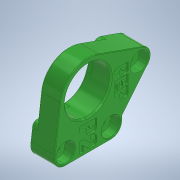
# Autodesk Inventor part: X-Axis Motor Support
Saved by Autodesk Inventor 2020 (Build 240168000, 168)
## iProperties
Created: 2019-09-17
Part Number: X-Axis Motor Support
Material: Generic
Document SubType Name: Modeling
Designer: pepd9
Density: 1 g/cm^3
Appearance: Smooth - Dark Forest Green
Author: pepd9
Autodesk Inventor part; units mm, degrees
ref_plane "YZ Plane" through (0, 0, 0) normal (1, 0, 0) x (0, 1, 0)
ref_plane "XZ Plane" through (0, 0, 0) normal (0, 1, 0) x (-1, 0, 0)
ref_plane "XY Plane" through (0, 0, 0) normal (0, 0, 1) x (1, 0, 0)
sketch "Sketch1" plane through (0, 0, 0) normal (1, 0, 0) x (0, 1, 0)
  circle A0 centre (0, 0) radius 8
  circle A1 centre (0, 0) radius 10
  dimension "d0" = 16
  dimension "d1" = 20
  constraints: 2 centre point, 2 coincident
  measures "d0" diameter of A0
  measures "d1" diameter of A1
extrude "Extrusion1" add sketch "Sketch1" along normal blind 6
sketch "Sketch2" plane through (0, 0, 0) normal (-1, 0, 0) x (0, 0, 1)
  circle A0 centre (0, 0) radius 8
  circle A1 centre (-18, 0) radius 2.75 construction
  circle A2 centre (-18, 0) radius 4
  circle A3 centre (0, 0) radius 10
  circle A4 centre (-18, 0) radius 1.5 construction
  line L0 (-19.5, 3.708099) -> (-3.736025, 9.275889)
  circle A5 centre (0, 0) radius 10
  line L1 (-12.888145, -9.569739) -> (-10.705089, -10.830127) construction
  line L2 (10.373932, -10.830127) -> (12.998008, -9.315116) construction
  circle A6 centre (-8, -15) radius 1.5 construction
  circle A7 centre (8, -15) radius 1.5 construction
  circle A8 centre (8, -15) radius 2.75 construction
  circle A9 centre (-8, -15) radius 2.75 construction
  circle A10 centre (-8, -15) radius 4
  circle A11 centre (8, -15) radius 4
  line L3 (-12, -15) -> (-12, -13.5)
  line L4 (11.832818, -13.855665) -> (9.920905, 1.255246)
  line L5 (8, -19) -> (-8, -19)
  line L6 (-12, -13.5) -> (-20.414736, -3.188895)
  point P0 (9.920905, 1.255246)
  point P1 (-3.736025, 9.275889)
  dimension "d4" = 5.5
  dimension "d5" = 8
  dimension "d6" = 18
  dimension "d7" = 3
  dimension "d8" = 3
  dimension "d9" = 3
  dimension "d10" = 5.5
  dimension "d11" = 5.5
  dimension "d12" = 8
  dimension "d13" = 8
  dimension "d14" = 15
  dimension "d15" = 8
  dimension "d16" = 8
  constraints: 10 end point, 9 centre point, 9 coincident, 8 point on circle, 2 tangent, 1 horizontal alignment, 1 vertical
  measures "d4" diameter of A1
  measures "d5" diameter of A2
  measures "d6" distance of point (0, 0) A1.centre
  measures "d7" diameter of A4
  measures "d8" diameter of A6
  measures "d9" diameter of A7
  measures "d10" diameter of A8
  measures "d11" diameter of A9
  measures "d12" diameter of A10
  measures "d13" diameter of A11
  measures "d14" vertical distance of A6.centre point (0, 0)
  measures "d15" horizontal distance of point (0, 0) A8.centre
  measures "d16" horizontal distance of point (0, 0) A6.centre
extrude "Extrusion2" add sketch "Sketch2" against normal blind 6 contours A2 | A2 L0 A3 L4 A11 L5 A10 L3 L6 | A10 | A11
sketch "Sketch3" plane through (6, 0, 0) normal (1, 0, 0) x (0, 0, -1)
  arc A0 (20.414736, -3.188895) -> (19.5, 3.708099) centre (18, 0) ccw
  arc A1 (8, -19) -> (12, -15) centre (8, -15) ccw
  arc A2 (-11.832818, -13.855665) -> (-8, -19) centre (-8, -15) ccw
  point P0 (0, 0)
hole "Hole1" at (6, 0, -18) at (6, -15, -8) at (6, -15, 8) direction (-1, 0, 0) diameter 3.2 end through all counterbore diameter 6.5 counterbore depth 2 clearance for "Socket Head Cap Screw" size "M3" standard "Ansi Metric M Profile"
sketch "Sketch4" plane through (6, 0, 0) normal (1, 0, 0) x (0, 0, -1)
  circle A0 centre (8, -15) radius 3.25
  circle A1 centre (18, 0) radius 3.25
  circle A2 centre (-8, -15) radius 3.25
  arc A3 (3.736025, 9.275889) -> (-9.920905, 1.255246) centre (0, 0) ccw
  line L0 (-9.920905, 1.255246) -> (-11.832818, -13.855665)
  arc A4 (-11.832818, -13.855665) -> (-8, -19) centre (-8, -15) ccw
  line L1 (-8, -19) -> (8, -19)
  arc A5 (8, -19) -> (12, -15) centre (8, -15) ccw
  line L2 (12, -15) -> (12, -13.5)
  line L3 (12, -13.5) -> (20.414736, -3.188895)
  arc A6 (20.414736, -3.188895) -> (19.5, 3.708099) centre (18, 0) ccw
  line L4 (19.5, 3.708099) -> (3.736025, 9.275889)
  circle A7 centre (0, 0) radius 8
  circle A8 centre (0, 0) radius 4
  dimension "d26" = 8
  constraints: 1 centre point, 1 coincident
  measures "d26" diameter of A8
extrude "Extrusion3" add sketch "Sketch4" along normal blind 1 contours L4 A6 L3 L2 A5 L1 A4 L0 A3 | A7
sketch "Sketch5" plane through (0, 0, 0) normal (-1, 0, 0) x (0, 0, 1)
  circle A0 centre (-8, -15) radius 1.6
  circle A1 centre (-18, 0) radius 1.6
  circle A2 centre (8, -15) radius 1.6
  arc A3 (9.920905, 1.255246) -> (-3.736025, 9.275889) centre (0, 0) ccw
  line L0 (-3.736025, 9.275889) -> (-19.5, 3.708099)
  arc A4 (-19.5, 3.708099) -> (-20.414736, -3.188895) centre (-18, 0) ccw
  line L1 (-20.414736, -3.188895) -> (-12, -13.5)
  line L2 (-12, -13.5) -> (-12, -15)
  arc A5 (-12, -15) -> (-8, -19) centre (-8, -15) ccw
  line L3 (-8, -19) -> (8, -19)
  arc A6 (8, -19) -> (11.832818, -13.855665) centre (8, -15) ccw
  line L4 (11.832818, -13.855665) -> (9.920905, 1.255246)
  circle A7 centre (0, 0) radius 8
  circle A8 centre (0, 0) radius 8
  line L5 (0, -8) -> (11.091928, -8)
  line L6 (11.832818, -13.855665) -> (9.920905, 1.255246)
  line L7 (-7.667515, -2.282371) -> (-10.979812, 6.717405)
  constraints: 4 end point, 2 point on circle, 2 point on line, 1 horizontal, 1 tangent
ref_plane "Work Plane1" through (-3.5, -20.915116, -29.665578) normal (1, 0, 0) x (0, 1, 0)
extrude "Extrusion4" add sketch "Sketch5" along normal blind 1.8 contours L4 A6 L3 A5 L2 L1 A4 L0 L7 A7 L5
fillet "Fillet1" radius 2 2 edges at (-0.9, -8, 11.0919) (-0.9, 6.7174, -10.9798)
chamfer "Chamfer1" distance 0.5 angle 45 13 edges at (-1.8, 0.5259, -21.9653) (-1.8, 4.8841, -16.1705) (-1.8, 5.9843, -11.3243) (-1.8, 1.2913, -8.9828) (-1.8, -6.4132, -4.7823) (-1.8, -8, 4.6645) (-1.8, -8.4997, 10.6515) (-1.8, -11.8023, 11.573) (-1.8, -17.3898, 11.2076) (-1.8, -19, 0) (-1.8, -17.8284, -10.8284) (-1.8, -14.25, -12) (-1.8, -8.3444, -16.2074)
chamfer "Chamfer2" distance 0.2 angle 45 12 edges at (7, 8.6229, 5.0642) (7, -6.3002, 10.8769) (7, 6.492, -11.618) (7, 0.5259, -21.9653) (7, -8.3444, -16.2074) (7, -17.8284, -10.8284) (7, -14.25, -12) (7, -19, 0) (7, -17.3898, 11.2076) (7, -15, 11.25) (7, 0, 4) (7, -15, -4.75)
chamfer "Chamfer3" distance 0.5 angle 45 5 edges at (0, -3.3724, 10.5064) (0, -8.8745, 11.2026) (0, 8.6229, 5.0642) (0, 7.9966, -7.3579) (0, 6.3887, -11.9104)
chamfer "Chamfer4" distance 0.5 angle 45 2 edges at (0, 4.7823, -6.4132) (0, 0, 8)
sketch "Sketch7" plane through (4, 0, -18) normal (1, 0, 0) x (0, 0, -1)
  circle A0 centre (0, 0) radius 3.25 projected
  circle A1 centre (0, 0) radius 1.6 projected
  circle A2 centre (-10, -15) radius 3.25 projected
  circle A3 centre (-10, -15) radius 1.6 projected
  circle A4 centre (-26, -15) radius 3.25 projected
  circle A5 centre (-26, -15) radius 1.6 projected
  line L0 (-3.25, 1.6) -> (3.25, 1.6)
  line L1 (3.25, 1.6) -> (3.25, -1.6)
  line L2 (3.25, -1.6) -> (-3.25, -1.6)
  line L3 (-3.25, -1.6) -> (-3.25, 1.6)
  line L4 (-3.25, 1.6) -> (3.25, -1.6) construction
  line L5 (3.25, 1.6) -> (-3.25, -1.6) construction
  line L6 (-13.25, -13.4) -> (-6.75, -13.4)
  line L7 (-6.75, -13.4) -> (-6.75, -16.6)
  line L8 (-6.75, -16.6) -> (-13.25, -16.6)
  line L9 (-13.25, -16.6) -> (-13.25, -13.4)
  line L10 (-13.25, -13.4) -> (-6.75, -16.6) construction
  line L11 (-6.75, -13.4) -> (-13.25, -16.6) construction
  line L12 (-29.25, -13.4) -> (-22.75, -13.4)
  line L13 (-22.75, -13.4) -> (-22.75, -16.6)
  line L14 (-22.75, -16.6) -> (-29.25, -16.6)
  line L15 (-29.25, -16.6) -> (-29.25, -13.4)
  line L16 (-29.25, -13.4) -> (-22.75, -16.6) construction
  line L17 (-22.75, -13.4) -> (-29.25, -16.6) construction
  point P0 (-18, 0)
  point P1 (-26, -16.6)
  point P2 (-23.171131, -16.6)
  point P3 (-23.171131, -13.4)
  point P4 (-26, -13.4)
  point P5 (-28.828869, -16.6)
  point P6 (-28.828869, -13.4)
  point P7 (-10, -16.6)
  point P8 (-7.171131, -16.6)
  point P9 (-7.171131, -13.4)
  point P10 (-10, -13.4)
  point P11 (-12.828869, -16.6)
  point P12 (-12.828869, -13.4)
  point P13 (-2.828869, -1.6)
  point P14 (0, -1.6)
  point P15 (0, 1.6)
  point P16 (-2.828869, 1.6)
  point P17 (2.828869, -1.6)
  point P18 (2.828869, 1.6)
  constraints: 36 end point, 6 midpoint, 6 parallel, 3 horizontal, 3 perpendicular
extrude "Extrusion6" cut sketch "Sketch7" against normal blind 0.4 contours A0 L2 A1 L0 | L0 A1 L2 A0 | A2 L8 A3 L6 | L6 A3 L8 A2 | A4 L14 A5 L12 | L12 A5 L14 A4
sketch "Sketch8" plane through (7, 0, 0) normal (1, 0, 0) x (0, 0, -1)
  circle A0 centre (0, 0) radius 8 projected
extrude "Extrusion7" cut sketch "Sketch8" against normal through all
chamfer "Chamfer5" distance 0.5 angle 45 1 edges at (7, 0, 8)
sketch "Sketch9" plane through (7, 0, 0) normal (1, 0, 0) x (0, 0, -1)
  line L0 (14.09513, 2.10245) -> (14.09513, -15.072793) construction
  line L1 (14.09513, -15.072793) -> (6.09513, -15.072793) construction
  line L2 (6.09513, -15.072793) -> (6.09513, 2.10245) construction
  line L3 (6.09513, 2.10245) -> (14.09513, 2.10245) construction
  line L4 (9.09513, 1.833994) -> (14.09513, 1.833994)
  line L5 (14.09513, 1.833994) -> (14.09513, -0.116043)
  spline S0 degree 2 poles (14.09513, -0.116043) (14.09513, -0.794642) (13.502289, -1.49934) (12.864705, -1.603739) knots 0 0 0 1 2 2 2
  spline S1 degree 2 poles (12.864705, -1.603739) (12.655906, -1.633568) (12.510492, -1.641025) (12.454563, -1.641025) knots 0 0 0 1 2 2 2
  spline S2 degree 2 poles (12.454563, -1.641025) (11.749865, -1.641025) (10.959411, -0.768542) (10.959411, 0.010728) knots 0 0 0 1 2 2 2
  line L6 (10.959411, 0.010728) -> (10.959411, 0.405955)
  line L7 (10.959411, 0.405955) -> (9.09513, 0.405955)
  line L8 (9.09513, 0.405955) -> (9.09513, 1.833994)
  spline S3 degree 2 poles (12.010865, 0.193427) (12.010865, 0.089027) (12.186107, -0.134686) (12.365078, -0.171972) knots 0 0 0 1 2 2 2
  spline S4 degree 2 poles (12.365078, -0.171972) (12.458292, -0.190615) (12.54032, -0.190615) knots 0 0 0 1 1 1
  spline S5 degree 2 poles (12.54032, -0.190615) (12.771491, -0.190615) (13.036219, 0.025642) (13.036219, 0.178513) knots 0 0 0 1 2 2 2
  line L9 (13.036219, 0.178513) -> (13.036219, 0.405955)
  line L10 (13.036219, 0.405955) -> (12.010865, 0.405955)
  line L11 (12.010865, 0.405955) -> (12.010865, 0.193427)
  line L12 (9.09513, -1.842367) -> (14.09513, -1.842367)
  line L13 (14.09513, -1.842367) -> (14.09513, -4.847587)
  line L14 (14.09513, -4.847587) -> (12.939276, -4.847587)
  line L15 (12.939276, -4.847587) -> (12.939276, -3.270406)
  line L16 (12.939276, -3.270406) -> (12.193564, -3.270406)
  line L17 (12.193564, -3.270406) -> (12.193564, -4.750645)
  line L18 (12.193564, -4.750645) -> (11.086182, -4.750645)
  line L19 (11.086182, -4.750645) -> (11.086182, -3.270406)
  line L20 (11.086182, -3.270406) -> (10.250984, -3.270406)
  line L21 (10.250984, -3.270406) -> (10.250984, -4.899787)
  line L22 (10.250984, -4.899787) -> (9.09513, -4.899787)
  line L23 (9.09513, -4.899787) -> (9.09513, -1.842367)
  line L24 (9.09513, -5.224172) -> (14.09513, -5.224172)
  line L25 (14.09513, -5.224172) -> (14.09513, -7.174209)
  spline S6 degree 2 poles (14.09513, -7.174209) (14.09513, -7.852807) (13.502289, -8.557505) (12.864705, -8.661905) knots 0 0 0 1 2 2 2
  spline S7 degree 2 poles (12.864705, -8.661905) (12.655906, -8.691733) (12.510492, -8.69919) (12.454563, -8.69919) knots 0 0 0 1 2 2 2
  spline S8 degree 2 poles (12.454563, -8.69919) (11.749865, -8.69919) (10.959411, -7.826707) (10.959411, -7.047438) knots 0 0 0 1 2 2 2
  line L26 (10.959411, -7.047438) -> (10.959411, -6.652211)
  line L27 (10.959411, -6.652211) -> (9.09513, -6.652211)
  line L28 (9.09513, -6.652211) -> (9.09513, -5.224172)
  spline S9 degree 2 poles (12.010865, -6.864738) (12.010865, -6.969138) (12.186107, -7.192852) (12.365078, -7.230137) knots 0 0 0 1 2 2 2
  spline S10 degree 2 poles (12.365078, -7.230137) (12.458292, -7.24878) (12.54032, -7.24878) knots 0 0 0 1 1 1
  spline S11 degree 2 poles (12.54032, -7.24878) (12.771491, -7.24878) (13.036219, -7.032524) (13.036219, -6.879653) knots 0 0 0 1 2 2 2
  line L29 (13.036219, -6.879653) -> (13.036219, -6.652211)
  line L30 (13.036219, -6.652211) -> (12.010865, -6.652211)
  line L31 (12.010865, -6.652211) -> (12.010865, -6.864738)
  point P0 (0, 0)
  constraints: 2 other
extrude "Extrusion8" cut sketch "Sketch9" against normal blind 0.6
sketch "Sketch10" plane through (7, 0, 0) normal (1, 0, 0) x (0, 0, -1)
  line L0 (3.056419, -9.325871) -> (3.056419, -19.630122) construction
  line L1 (3.056419, -19.630122) -> (-4.027101, -19.630122) construction
  line L2 (-4.027101, -19.630122) -> (-4.027101, -9.325871) construction
  line L3 (-4.027101, -9.325871) -> (3.056419, -9.325871) construction
  line L4 (-3.01517, -9.648019) -> (2.984831, -9.648019)
  line L5 (2.984831, -9.648019) -> (2.984831, -11.988064)
  spline S0 degree 2 poles (2.984831, -11.988064) (2.984831, -12.802381) (2.273421, -13.648019) (1.50832, -13.773298) knots 0 0 0 1 2 2 2
  spline S1 degree 2 poles (1.50832, -13.773298) (1.257761, -13.809093) (1.083264, -13.818041) (1.01615, -13.818041) knots 0 0 0 1 2 2 2
  spline S2 degree 2 poles (1.01615, -13.818041) (0.170513, -13.818041) (-0.778033, -12.771061) (-0.778033, -11.835938) knots 0 0 0 1 2 2 2
  line L6 (-0.778033, -11.835938) -> (-0.778033, -11.361665)
  line L7 (-0.778033, -11.361665) -> (-3.01517, -11.361665)
  line L8 (-3.01517, -11.361665) -> (-3.01517, -9.648019)
  spline S3 degree 2 poles (0.483712, -11.616699) (0.483712, -11.741979) (0.694003, -12.010435) (0.908768, -12.055178) knots 0 0 0 1 2 2 2
  spline S4 degree 2 poles (0.908768, -12.055178) (1.020625, -12.077549) (1.119059, -12.077549) knots 0 0 0 1 1 1
  spline S5 degree 2 poles (1.119059, -12.077549) (1.396464, -12.077549) (1.714137, -11.818041) (1.714137, -11.634596) knots 0 0 0 1 2 2 2
  line L9 (1.714137, -11.634596) -> (1.714137, -11.361665)
  line L10 (1.714137, -11.361665) -> (0.483712, -11.361665)
  line L11 (0.483712, -11.361665) -> (0.483712, -11.616699)
  spline S6 degree 2 poles (-3.01517, -13.997012) (-2.514051, -13.997012) (-1.838436, -14.122292) (-1.498391, -14.296788) knots 0 0 0 1 2 2 2
  spline S7 degree 2 poles (-1.498391, -14.296788) (-1.194141, -14.439965) (-0.710919, -14.833701) (-0.330606, -15.227437) knots 0 0 0 1 2 2 2
  line L12 (-0.330606, -15.227437) -> (0.152616, -15.697236)
  spline S8 degree 2 poles (0.152616, -15.697236) (0.613466, -16.108869) (1.011676, -16.310211) (1.347247, -16.310211) knots 0 0 0 1 2 2 2
  spline S9 degree 2 poles (1.347247, -16.310211) (1.463578, -16.310211) (1.620177, -16.28784) (1.69624, -16.25652) knots 0 0 0 1 2 2 2
  spline S10 degree 2 poles (1.69624, -16.25652) (1.924428, -16.158086) (1.924428, -15.974641) knots 0 0 0 1 1 1
  spline S11 degree 2 poles (1.924428, -15.974641) (1.924428, -15.934372) (1.866262, -15.755401) (1.553063, -15.621173) (1.168276, -15.621173) knots 0 0 0 1 2 3 3 3
  line L13 (1.168276, -15.621173) -> (0.908768, -15.621173)
  line L14 (0.908768, -15.621173) -> (0.908768, -14.019384)
  line L15 (0.908768, -14.019384) -> (1.213018, -14.014909)
  spline S12 degree 2 poles (1.213018, -14.014909) (1.825994, -14.014909) (2.573197, -14.408645) (2.819282, -14.865021) knots 0 0 0 1 2 2 2
  spline S13 degree 2 poles (2.819282, -14.865021) (2.962459, -15.129003) (3.056419, -15.844887) (3.056419, -16.082023) knots 0 0 0 1 2 2 2
  spline S14 degree 2 poles (3.056419, -16.082023) (3.056419, -16.909764) (2.353958, -17.831464) (1.682817, -17.938847) knots 0 0 0 1 2 2 2
  spline S15 degree 2 poles (1.682817, -17.938847) (1.284607, -18.005961) (1.04747, -18.005961) knots 0 0 0 1 1 1
  spline S16 degree 2 poles (1.04747, -18.005961) (0.707426, -18.005961) (0.197358, -17.777773) (-0.151635, -17.495894) knots 0 0 0 1 2 2 2
  line L16 (-0.151635, -17.495894) -> (-1.189666, -16.489182)
  line L17 (-1.189666, -16.489182) -> (-1.292575, -16.377325)
  line L18 (-1.292575, -16.377325) -> (-1.50734, -16.189406)
  line L19 (-1.50734, -16.189406) -> (-1.614722, -16.095446)
  line L20 (-1.614722, -16.095446) -> (-1.654991, -16.064126)
  line L21 (-1.654991, -16.064126) -> (-1.686311, -15.988064)
  line L22 (-1.686311, -15.988064) -> (-1.686311, -17.947795)
  line L23 (-1.686311, -17.947795) -> (-3.01517, -17.947795)
  line L24 (-3.01517, -17.947795) -> (-3.01517, -13.997012)
  point P0 (0, 0)
  constraints: 2 other
extrude "Extrusion9" cut sketch "Sketch10" against normal blind 0.6
body "Solid1"
